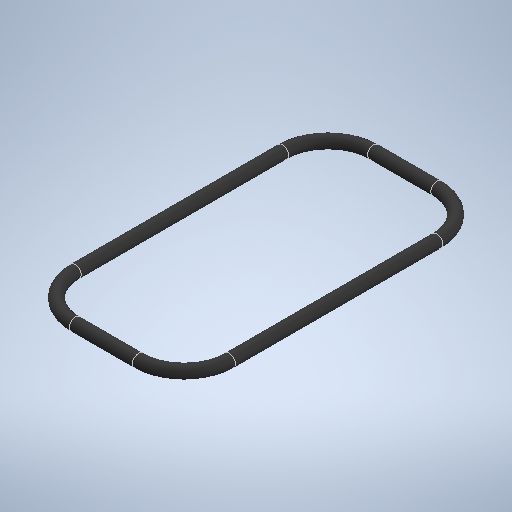
# Autodesk Inventor part: o-ring installed
Saved by Autodesk Inventor 2025 (Build 290162000, 162)
## iProperties
Created: 2024-05-14
Part Number: o-ring installed
Material: Rubber
Document SubType Name: Modeling
Designer: Caleb Fangmeier
Density: 0.93 g/cm^3
Appearance: Rubber - Black
Author: Caleb Fangmeier
Autodesk Inventor part; units mm, degrees
ref_plane "YZ Plane" through (0, 0, 0) normal (1, 0, 0) x (0, 1, 0)
ref_plane "XZ Plane" through (0, 0, 0) normal (0, 1, 0) x (-1, 0, 0)
ref_plane "XY Plane" through (0, 0, 0) normal (0, 0, 1) x (1, 0, 0)
sketch "Sketch1" plane through (0, 0, 0) normal (0, 1, 0) x (-1, 0, 0)
  line L0 (-3.125, -14.75) -> (3.125, -14.75)
  line L1 (7.625, -10.25) -> (7.625, 10.25)
  line L2 (3.125, 14.75) -> (-3.125, 14.75)
  line L3 (-7.625, 10.25) -> (-7.625, -10.25)
  line L4 (-7.625, -14.75) -> (7.625, 14.75) construction
  line L5 (7.625, -14.75) -> (-7.625, 14.75) construction
  arc A0 (7.625, 10.25) -> (3.125, 14.75) centre (3.125, 10.25) ccw
  arc A1 (-3.125, 14.75) -> (-7.625, 10.25) centre (-3.125, 10.25) ccw
  arc A2 (-7.625, -10.25) -> (-3.125, -14.75) centre (-3.125, -10.25) ccw
  arc A3 (3.125, -14.75) -> (7.625, -10.25) centre (3.125, -10.25) ccw
  point P0 (0, 0)
  dimension "d0" = 29.5
  dimension "d1" = 15.25
  dimension "d2" = 4.5
  constraints: 12 end point, 8 point on circle, 8 point on line, 8 tangent, 4 centre point, 3 equal radius, 2 midpoint, 2 parallel, 1 horizontal, 1 perpendicular
  measures "d0" distance of L5.start L4.end
  measures "d1" distance of L4.end L5.end
  measures "d2" radius of A0
sketch "Sketch2" plane through (0, 0, 0) normal (0, 0, 1) x (1, 0, 0)
  line L0 (7.625, 0) -> (-7.625, 0) construction
  line L1 (-7.625, 0) -> (7.625, 0) construction
  line L2 (7.625, 0) -> (3.125, 0) projected
  line L3 (7.625, 0) -> (3.125, 0) projected
  circle A0 centre (7.625, 0) radius 0.6
  point P0 (0, 0)
  point P1 (7.625, 0)
  point P2 (7.625, 0)
  dimension "d3" = 1.2
  constraints: 1 centre point, 1 coincident, 1 other
  measures "d3" diameter of A0
sweep "Sweep1" add profiles "Sketch2" path "Sketch1" path curves L3 A2 L0 A3 L1 A0 L2 A1
body "Solid1"
